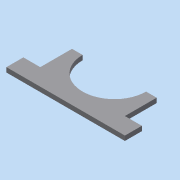
# Autodesk Inventor part: anillo5
Saved by Autodesk Inventor 2015 (Build 190159000, 159)
## iProperties
Created: 2017-09-29
Part Number: anillo5
Material: Generic
Document SubType Name: Modeling
Designer: macbook
Density: 1 g/cm^3
Appearance: Default
Author: macbook
Autodesk Inventor part; units mm, degrees
ref_plane "YZ Plane" through (0, 0, 0) normal (1, 0, 0) x (0, 1, 0)
ref_plane "XZ Plane" through (0, 0, 0) normal (0, 1, 0) x (-1, 0, 0)
ref_plane "XY Plane" through (0, 0, 0) normal (0, 0, 1) x (1, 0, 0)
sketch "Sketch1" plane through (0, 0, 0) normal (0, 0, 1) x (1, 0, 0)
  line L0 (0, 170) -> (100, 170)
  circle A0 centre (50, 207.5) radius 37.5
  line L1 (100, 150) -> (0, 150)
  line L2 (120, 170) -> (-20, 170)
  line L3 (100, 170) -> (100, 207.5)
  line L4 (100, 207.5) -> (87.5, 207.5)
  line L5 (0, 170) -> (0, 207.5)
  line L6 (0, 207.5) -> (12.5, 207.5)
  line L7 (-20, 170) -> (-20, 150)
  line L8 (-20, 150) -> (0, 150)
  line L9 (100, 150) -> (120, 150)
  line L10 (120, 150) -> (120, 170)
  point P0 (0, 0)
  dimension "d0" = 75
  dimension "d1" = 140
  constraints: 22 end point, 4 perpendicular, 3 vertical, 2 point on circle, 2 point on line, 1 centre point, 1 horizontal
  measures "d0" diameter of A0
  measures "d1" distance of L2.end L2.start
extrude "Extrusion1" add sketch "Sketch1" along normal blind 5.5 contours L5 L6 A0 L0 | L0 L2 L10 L9 L1 L8 L7 | A0 L4 L3 L0
body "Solid1"
